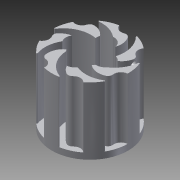
# Autodesk Inventor part: Mecanum Adapter print
Saved by Autodesk Inventor 2015 (Build 190159000, 159)
## iProperties
Created: 2016-09-13
Part Number: Mecanum Adapter print
Material: PC/ABS Plastic
Document SubType Name: Modeling
Designer: Eduardo
Density: 0.357273 g/cm^3
Appearance: Smooth - White
Author: Eduardo
Autodesk Inventor part; units mm, degrees
ref_plane "YZ Plane" through (0, 0, 0) normal (1, 0, 0) x (0, 1, 0)
ref_plane "XZ Plane" through (0, 0, 0) normal (0, 1, 0) x (-1, 0, 0)
ref_plane "XY Plane" through (0, 0, 0) normal (0, 0, 1) x (1, 0, 0)
sketch "Sketch1" plane through (0, 0, 0) normal (0, 1, 0) x (-1, 0, 0)
  arc A0 (16.3931, 7.8064) -> (15.4281, 8.9517) centre (9.359, 2.8585) ccw
  arc A1 (16.4388, 8.0888) -> (19.6285, 14.7315) centre (11.7364, 14.4339) ccw
  arc A2 (16.4388, 8.0888) -> (15.6268, 9.0387) centre (9.359, 2.8585) ccw
  arc A3 (15.6268, 9.0387) -> (6.1294, 21.905) centre (1.2891, 8.3936) ccw
  arc A4 (14.0341, 22.1773) -> (6.1816, 22.4793) centre (9.359, 2.8585) ccw
  arc A5 (14.0341, 22.1773) -> (17.423, 17.8969) centre (17.6894, 21.5896) ccw
  arc A6 (19.5396, 15.8747) -> (17.423, 17.8969) centre (17.2577, 15.6052) ccw
  arc A7 (19.6285, 14.7315) -> (19.5396, 15.8747) centre (5.281, 14.1906) ccw
  circle A8 centre (9.359, 2.8585) radius 8.6
  arc A9 (6.1816, 22.4793) -> (6.1294, 21.905) centre (6.2292, 22.1855) ccw
  arc A10 (9.684, 11.6547) -> (6.4792, 18.2902) centre (1.7912, 11.9343) ccw
  arc A11 (9.684, 11.6547) -> (8.4351, 11.6121) centre (9.359, 2.8585) ccw
  arc A12 (8.4351, 11.6121) -> (-7.5458, 12.2088) centre (-0.0001, 0.0002) ccw
  arc A13 (-2.8302, 18.5586) -> (-7.9622, 12.6077) centre (9.359, 2.8585) ccw
  arc A14 (-2.8302, 18.5586) -> (2.6293, 18.5395) centre (-0.0917, 21.0501) ccw
  arc A15 (5.53, 18.9334) -> (2.6293, 18.5395) centre (4.318, 16.9813) ccw
  arc A16 (6.4792, 18.2902) -> (5.53, 18.9334) centre (-2.0434, 6.7356) ccw
  arc A17 (-7.9622, 12.6077) -> (-7.5458, 12.2088) centre (-7.7029, 12.4617) ccw
  arc A18 (2.6844, 8.5969) -> (-4.5015, 10.2285) centre (-2.4552, 2.6004) ccw
  arc A19 (2.6844, 8.5969) -> (1.9391, 7.5939) centre (9.359, 2.8585) ccw
  arc A20 (1.9391, 7.5939) -> (-8.4914, -4.5284) centre (5.7584, -6.2409) ccw
  arc A21 (-10.5157, 3.1174) -> (-9.0628, -4.6053) centre (9.359, 2.8585) ccw
  arc A22 (-10.5157, 3.1174) -> (-7.0968, 7.3739) centre (-10.7561, 6.8119) ccw
  arc A23 (-5.5962, 9.8874) -> (-7.0968, 7.3739) centre (-4.8257, 7.7227) ccw
  arc A24 (-4.5015, 10.2285) -> (-5.5962, 9.8874) centre (-0.7815, -3.639) ccw
  arc A25 (-9.0628, -4.6053) -> (-8.4914, -4.5284) centre (-8.787, -4.4936) ccw
  arc A26 (0.711, 1.2179) -> (-5.045, -3.383) centre (2.1947, -6.5392) ccw
  arc A27 (0.711, 1.2179) -> (1.0305, 0.0098) centre (9.359, 2.8585) ccw
  arc A28 (1.0305, 0.0098) -> (4.0048, -15.7032) centre (14.2282, -5.63) ccw
  arc A29 (-3.2351, -12.5188) -> (3.7086, -16.1979) centre (9.359, 2.8585) ccw
  arc A30 (-3.2351, -12.5188) -> (-4.4313, -7.1919) centre (-6.2735, -10.4033) ccw
  arc A31 (-5.4608, -4.4515) -> (-4.4313, -7.1919) centre (-3.288, -5.1988) ccw
  arc A32 (-5.045, -3.383) -> (-5.4608, -4.4515) centre (8.1164, -9.1208) ccw
  arc A33 (3.7086, -16.1979) -> (4.0048, -15.7032) centre (3.7932, -15.9125) ccw
  arc A34 (5.2497, -4.9257) -> (5.2581, -12.2945) centre (12.2395, -8.6022) ccw
  arc A35 (5.2497, -4.9257) -> (6.3934, -5.4292) centre (9.359, 2.8585) ccw
  arc A36 (6.3934, -5.4292) -> (20.5328, -12.9006) centre (19.0314, 1.3729) ccw
  arc A37 (13.5291, -16.5756) -> (20.7349, -13.4407) centre (9.359, 2.8585) ccw
  arc A38 (13.5291, -16.5756) -> (8.6186, -14.1895) centre (9.9808, -17.6321) ccw
  arc A39 (5.8342, -13.2859) -> (8.6186, -14.1895) centre (7.7731, -12.053) ccw
  arc A40 (5.2581, -12.2945) -> (5.8342, -13.2859) centre (17.9501, -5.582) ccw
  arc A41 (20.7349, -13.4407) -> (20.5328, -12.9006) centre (20.5646, -13.1966) ccw
  arc A42 (12.8828, -5.2077) -> (18.6492, -9.7955) centre (20.1153, -2.0351) ccw
  arc A43 (12.8828, -5.2077) -> (13.9895, -4.6274) centre (9.359, 2.8585) ccw
  arc A44 (13.9895, -4.6274) -> (28.6467, 1.7688) centre (16.5512, 9.4944) ccw
  arc A45 (27.1532, -5.9982) -> (29.195, 1.5902) centre (9.359, 2.8585) ccw
  arc A46 (27.1532, -5.9982) -> (22.226, -8.3497) centre (25.7669, -9.4311) ccw
  arc A47 (19.7835, -9.9632) -> (22.226, -8.3497) centre (20.0285, -7.6786) ccw
  arc A48 (18.6492, -9.7955) -> (19.7835, -9.9632) centre (21.3145, 4.3127) ccw
  arc A49 (29.195, 1.5902) -> (28.6467, 1.7688) centre (28.8979, 1.6092) ccw
  arc A50 (17.8625, 0.5843) -> (25.0447, 2.2322) centre (19.8914, 8.217) ccw
  arc A51 (17.8625, 0.5843) -> (18.0988, 1.8114) centre (9.359, 2.8585) ccw
  arc A52 (18.0988, 1.8114) -> (22.2366, 17.2588) centre (8.6551, 12.6189) ccw
  arc A53 (27.3779, 11.2485) -> (22.7181, 17.5761) centre (9.359, 2.8585) ccw
  arc A54 (27.3779, 11.2485) -> (26.1444, 5.9301) centre (29.1975, 8.0242) ccw
  arc A55 (25.883, 3.0145) -> (26.1444, 5.9301) centre (24.2495, 4.6305) ccw
  arc A56 (25.0447, 2.2322) -> (25.883, 3.0145) centre (15.6762, 13.1123) ccw
  arc A57 (22.7181, 17.5761) -> (22.2366, 17.2588) centre (22.5181, 17.3557) ccw
  point P0 (0, 0)
  point P1 (8.3792, 11.4025)
  point P2 (2.0681, 7.4195)
  point P3 (1.2473, 0.002)
  point P4 (6.5348, -5.2646)
  point P5 (13.949, -4.4143)
  point P6 (17.9069, 1.9126)
  dimension "d2" = 360
  constraints: 114 point on circle, 58 centre point, 1 coincident, 1 concentric, 178 other
extrude "Extrusion1" add sketch "Sketch1" along normal blind 31.75 contours A2 A3 A9 A4 A5 A6 A7 A1 | A11 A12 A17 A13 A14 A15 A16 A10 | A19 A20 A25 A21 A22 A23 A24 A18 | A27 A28 A33 A29 A30 A31 A32 A26 | A35 A36 A41 A37 A38 A39 A40 A34 | A43 A44 A49 A45 A46 A47 A48 A42 | A51 A52 A57 A53 A54 A55 A56 A50
sketch "Sketch2" plane through (0, 0, 0) normal (0, -1, 0) x (1, 0, 0)
  arc A0 (-22.7181, 17.5761) -> (-27.3779, 11.2485) centre (-9.359, 2.8585) ccw projected
  arc A1 (-29.195, 1.5902) -> (-27.1532, -5.9982) centre (-9.359, 2.8585) ccw projected
  arc A2 (-20.7349, -13.4407) -> (-13.5291, -16.5756) centre (-9.359, 2.8585) ccw projected
  arc A3 (-3.7086, -16.1979) -> (3.2351, -12.5188) centre (-9.359, 2.8585) ccw projected
  circle A4 centre (-9.359, 2.8585) radius 19.8764
  point P0 (0, 0)
  point P1 (-9.359, 2.8585)
  constraints: 1 centre point, 1 coincident
extrude "Extrusion2" add sketch "Sketch2" along normal blind 3.175
sketch "Sketch3" plane through (-9.359, -3.175, 2.8585) normal (0, -1, 0) x (1, 0, 0)
  circle A0 centre (0, 0) radius 19.8764 projected
  arc A1 (0, 6.645) -> (0, 9.355) centre (0, 8) ccw
  arc A2 (0, 9.355) -> (0, 6.645) centre (0, 8) ccw
  arc A3 (-8, -1.355) -> (-8, 1.355) centre (-8, 0) ccw
  arc A4 (-8, 1.355) -> (-8, -1.355) centre (-8, 0) ccw
  arc A5 (8, 1.355) -> (8, -1.355) centre (8, 0) ccw
  arc A6 (8, -1.355) -> (8, 1.355) centre (8, 0) ccw
  arc A7 (0, -9.355) -> (0, -6.645) centre (0, -8) ccw
  arc A8 (0, -6.645) -> (0, -9.355) centre (0, -8) ccw
  arc A9 (0, 3.95) -> (0, -3.95) centre (0, 0) ccw
  arc A10 (0, -3.95) -> (0, 3.95) centre (0, 0) ccw
  circle A11 centre (0, 0) radius 3.975
  point P0 (9.359, -2.8585)
  dimension "d8" = 7.95
  constraints: 20 point on circle, 11 centre point, 1 coincident, 1 concentric
  measures "d8" diameter of A11
extrude "Extrusion3" cut sketch "Sketch3" against normal blind 50.8 contours A2 A1 | A4 A3 | A6 A5 | A8 A7 | A10 A9 | A11
sketch "Sketch4" plane through (0, 0, 0) normal (0, 1, 0) x (1, 0, 0)
  circle A0 centre (-1.359, -2.8585) radius 1.355 projected
  circle A1 centre (-9.359, 5.1415) radius 1.355 projected
  circle A2 centre (-9.359, -2.8585) radius 3.975 projected
  arc A3 (-12.8828, 5.2077) -> (-13.9895, 4.6274) centre (-9.359, -2.8585) ccw projected
  arc A4 (-13.9895, 4.6274) -> (-28.6467, -1.7688) centre (-16.5512, -9.4944) ccw projected
  arc A5 (-29.195, -1.5902) -> (-28.6467, -1.7688) centre (-28.8979, -1.6092) ccw projected
  arc A6 (-29.195, -1.5902) -> (-27.3779, -11.2485) centre (-9.359, -2.8585) ccw projected
  arc A7 (-27.3779, -11.2485) -> (-22.7181, -17.5761) centre (-9.359, -2.8585) ccw projected
  arc A8 (-22.7181, -17.5761) -> (-14.0341, -22.1773) centre (-9.359, -2.8585) ccw projected
  arc A9 (-14.0341, -22.1773) -> (-6.1816, -22.4793) centre (-9.359, -2.8585) ccw projected
  arc A10 (-6.1816, -22.4793) -> (2.8302, -18.5586) centre (-9.359, -2.8585) ccw projected
  arc A11 (2.8302, -18.5586) -> (7.9622, -12.6077) centre (-9.359, -2.8585) ccw projected
  arc A12 (7.9622, -12.6077) -> (10.5157, -3.1174) centre (-9.359, -2.8585) ccw projected
  arc A13 (10.5157, -3.1174) -> (9.0628, 4.6053) centre (-9.359, -2.8585) ccw projected
  arc A14 (9.0628, 4.6053) -> (3.2351, 12.5188) centre (-9.359, -2.8585) ccw projected
  arc A15 (3.2351, 12.5188) -> (-3.7086, 16.1979) centre (-9.359, -2.8585) ccw projected
  arc A16 (-3.7086, 16.1979) -> (-13.5291, 16.5756) centre (-9.359, -2.8585) ccw projected
  arc A17 (-13.5291, 16.5756) -> (-20.7349, 13.4407) centre (-9.359, -2.8585) ccw projected
  arc A18 (-20.7349, 13.4407) -> (-27.1532, 5.9982) centre (-9.359, -2.8585) ccw projected
  arc A19 (-27.1532, 5.9982) -> (-22.226, 8.3497) centre (-25.7669, 9.4311) ccw projected
  arc A20 (-19.7835, 9.9632) -> (-22.226, 8.3497) centre (-20.0285, 7.6786) ccw projected
  arc A21 (-18.6492, 9.7955) -> (-19.7835, 9.9632) centre (-21.3145, -4.3127) ccw projected
  arc A22 (-12.8828, 5.2077) -> (-18.6492, 9.7955) centre (-20.1153, 2.0351) ccw projected
  arc A23 (-27.1532, 5.9982) -> (-29.195, -1.5902) centre (-9.359, -2.8585) ccw projected
  arc A24 (-27.3779, -11.2485) -> (-26.1444, -5.9301) centre (-29.1975, -8.0242) ccw projected
  arc A25 (-25.883, -3.0145) -> (-26.1444, -5.9301) centre (-24.2495, -4.6305) ccw projected
  arc A26 (-25.0447, -2.2322) -> (-25.883, -3.0145) centre (-15.6762, -13.1123) ccw projected
  arc A27 (-17.8625, -0.5843) -> (-25.0447, -2.2322) centre (-19.8914, -8.217) ccw projected
  arc A28 (-17.8625, -0.5843) -> (-18.0868, -1.7155) centre (-9.359, -2.8585) ccw projected
  arc A29 (-18.0868, -1.7155) -> (-18.5615, -2.2338) centre (-17.359, -2.8585) ccw projected
  arc A30 (-18.5615, -2.2338) -> (-22.2366, -17.2588) centre (-8.6551, -12.6189) ccw projected
  arc A31 (-22.7181, -17.5761) -> (-22.2366, -17.2588) centre (-22.5181, -17.3557) ccw projected
  arc A32 (-14.0341, -22.1773) -> (-17.423, -17.8969) centre (-17.6894, -21.5896) ccw projected
  arc A33 (-19.5396, -15.8747) -> (-17.423, -17.8969) centre (-17.2577, -15.6052) ccw projected
  arc A34 (-19.6285, -14.7315) -> (-19.5396, -15.8747) centre (-5.281, -14.1906) ccw projected
  arc A35 (-16.4388, -8.0888) -> (-19.6285, -14.7315) centre (-11.7364, -14.4339) ccw projected
  arc A36 (-16.4388, -8.0888) -> (-15.6268, -9.0387) centre (-9.359, -2.8585) ccw projected
  arc A37 (-15.6268, -9.0387) -> (-6.1294, -21.905) centre (-1.2891, -8.3936) ccw projected
  arc A38 (-6.1816, -22.4793) -> (-6.1294, -21.905) centre (-6.2292, -22.1855) ccw projected
  arc A39 (2.8302, -18.5586) -> (-2.6293, -18.5395) centre (0.0917, -21.0501) ccw projected
  arc A40 (-5.53, -18.9334) -> (-2.6293, -18.5395) centre (-4.318, -16.9813) ccw projected
  arc A41 (-6.4792, -18.2902) -> (-5.53, -18.9334) centre (2.0434, -6.7356) ccw projected
  arc A42 (-9.6853, -12.1736) -> (-6.4792, -18.2902) centre (-1.7912, -11.9343) ccw projected
  arc A43 (-9.6853, -12.1736) -> (-8.3027, -11.7071) centre (-9.359, -10.8585) ccw projected
  arc A44 (-8.3027, -11.7071) -> (7.5458, -12.2088) centre (0.0001, -0.0002) ccw projected
  arc A45 (7.9622, -12.6077) -> (7.5458, -12.2088) centre (7.7029, -12.4617) ccw projected
  arc A46 (10.5157, -3.1174) -> (7.0968, -7.3739) centre (10.7561, -6.8119) ccw projected
  arc A47 (5.5962, -9.8874) -> (7.0968, -7.3739) centre (4.8257, -7.7227) ccw projected
  arc A48 (4.5015, -10.2285) -> (5.5962, -9.8874) centre (0.7815, 3.639) ccw projected
  arc A49 (-2.6844, -8.5969) -> (4.5015, -10.2285) centre (2.4552, -2.6004) ccw projected
  arc A50 (-2.6844, -8.5969) -> (-1.9391, -7.5939) centre (-9.359, -2.8585) ccw projected
  arc A51 (-1.9391, -7.5939) -> (8.4914, 4.5284) centre (-5.7584, 6.2409) ccw projected
  arc A52 (9.0628, 4.6053) -> (8.4914, 4.5284) centre (8.787, 4.4936) ccw projected
  arc A53 (3.2351, 12.5188) -> (4.4313, 7.1919) centre (6.2735, 10.4033) ccw projected
  arc A54 (5.4608, 4.4515) -> (4.4313, 7.1919) centre (3.288, 5.1988) ccw projected
  arc A55 (5.045, 3.383) -> (5.4608, 4.4515) centre (-8.1164, 9.1208) ccw projected
  arc A56 (-0.711, -1.2179) -> (5.045, 3.383) centre (-2.1947, 6.5392) ccw projected
  arc A57 (-0.711, -1.2179) -> (-1.0305, -0.0098) centre (-9.359, -2.8585) ccw projected
  arc A58 (-1.0305, -0.0098) -> (-4.0048, 15.7032) centre (-14.2282, 5.63) ccw projected
  arc A59 (-3.7086, 16.1979) -> (-4.0048, 15.7032) centre (-3.7932, 15.9125) ccw projected
  arc A60 (-13.5291, 16.5756) -> (-8.6186, 14.1895) centre (-9.9808, 17.6321) ccw projected
  arc A61 (-5.8342, 13.2859) -> (-8.6186, 14.1895) centre (-7.7731, 12.053) ccw projected
  arc A62 (-5.2581, 12.2945) -> (-5.8342, 13.2859) centre (-17.9501, 5.582) ccw projected
  arc A63 (-5.2497, 4.9257) -> (-5.2581, 12.2945) centre (-12.2395, 8.6022) ccw projected
  arc A64 (-5.2497, 4.9257) -> (-6.3934, 5.4292) centre (-9.359, -2.8585) ccw projected
  arc A65 (-6.3934, 5.4292) -> (-20.5328, 12.9006) centre (-19.0314, -1.3729) ccw projected
  arc A66 (-20.7349, 13.4407) -> (-20.5328, 12.9006) centre (-20.5646, 13.1966) ccw projected
  arc A67 (-18.5615, -2.2338) -> (-18.0868, -1.7155) centre (-17.359, -2.8585) ccw projected
  arc A68 (-8.3027, -11.7071) -> (-9.6853, -12.1736) centre (-9.359, -10.8585) ccw projected
  circle A69 centre (-9.359, -10.8585) radius 4.585
  circle A70 centre (-9.359, -2.8585) radius 3.975
  circle A71 centre (-1.359, -2.8585) radius 4.585
  circle A72 centre (-9.359, 5.1415) radius 4.585
  circle A73 centre (-17.359, -2.8585) radius 4.585
  point P0 (0, 0)
  dimension "d11" = 9.17
  dimension "d14" = 360
  constraints: 5 centre point, 2 coincident, 1 concentric, 9 other
  measures "d11" diameter of A69
extrude "Extrusion4" cut sketch "Sketch4" along normal blind 101.6 contours A2 A71 | A2 A71 A58 A57 A56 A51 | A72 A2 | A2 A72 A3 A22 A65 A64 A63 | A71 A56 A57 A58 | A69 A44 A68 A42 A2 | A2 A69 | A51 A71 | A73 A2 | A2 A73 A30 A67 A28 A27 | A72 A22 A3 | A63 A64 A65 A72 | A42 A43 A44 A69 | A27 A28 A29 A30 A73
sketch "Sketch5" plane through (0, 0, 0) normal (1, 0, 0) x (0, 1, 0)
  line L0 (-3.175, -14.6767) -> (-3.175, 20.3936) projected
  line L1 (-3.175, 20.3936) -> (0, 20.3936) projected
  line L2 (0, 20.3936) -> (0, 17.3489) projected
  line L3 (0, 17.3489) -> (31.75, 17.3489) projected
  line L4 (31.75, 17.3489) -> (31.75, 14.3525) projected
  line L5 (31.75, 14.3525) -> (0, 14.3525) projected
  line L6 (0, 14.3525) -> (0, 10.1068) projected
  line L7 (0, 10.1068) -> (31.75, 10.1068) projected
  line L8 (31.75, 10.1068) -> (31.75, 7.2374) projected
  line L9 (31.75, 7.2374) -> (0, 7.2374) projected
  line L10 (0, 7.2374) -> (0, -1.5205) projected
  line L11 (0, -1.5205) -> (31.75, -1.5205) projected
  line L12 (31.75, -1.5205) -> (31.75, -3.7469) projected
  line L13 (31.75, -3.7469) -> (0, -3.7469) projected
  line L14 (0, -3.7469) -> (0, -7.513) projected
  line L15 (0, -7.513) -> (31.75, -7.513) projected
  line L16 (31.75, -7.513) -> (31.75, -14.6767) projected
  line L17 (31.75, -14.6767) -> (-3.175, -14.6767) projected
  line L18 (31.75, -1.6342) -> (31.75, -15.7032) projected
  circle A0 centre (28.8798, -5.6265) radius 1.753
  point P0 (0, 0)
  dimension "d18" = 3.506
  dimension "d20" = 2.8702
  dimension "d21" = 1.8796
  constraints: 1 centre point
  measures "d18" diameter of A0
  measures "d20" distance from line of L18 A0.centre
  measures "d21" distance from line of A0.centre L13
extrude "Extrusion5" cut sketch "Sketch5" along normal blind 6.35 contours A0
body "Solid1"
